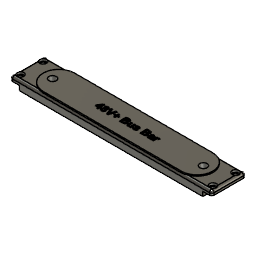
Compartment Mount (Autodesk Fusion 360 archive; units mm, degrees)
design "Upper Platform"
part number: 2026-01-22-12-11-46-373
Autodesk Fusion 360 part; units mm, degrees
sketch "Base" plane through (0, 0, 0) normal (0, 0, 1) x (1, 0, 0)
  line L0 (89, 15) -> (-89, 15)
  line L1 (-89, 15) -> (-89, -15)
  line L2 (-89, -15) -> (89, -15)
  line L3 (89, -15) -> (89, 15)
  line L4 (89, 15) -> (-89, -15) construction
  line L5 (-89, 15) -> (89, -15) construction
  line L6 (81, 15) -> (-81, 15)
  line L7 (-81, 15) -> (-81, -15)
  line L8 (-81, -15) -> (81, -15)
  line L9 (81, -15) -> (81, 15)
  line L10 (81, 15) -> (-81, -15) construction
  line L11 (-81, 15) -> (81, -15) construction
  dimension "d1" = 178
  dimension "d2" = 30
  dimension "d3" = 162
  constraint horizontal L0
  constraint perpendicular L0 L1
  constraint parallel L0 L2
  constraint parallel L1 L3
  constraint coincident L4 origin
  constraint coincident L5 origin
  constraint horizontal L6
  constraint perpendicular L6 L7
  constraint parallel L6 L8
  constraint parallel L7 L9
  constraint coincident L10 origin
  constraint coincident L11 origin
  measures "d1" distance of L1.end L2.end
  measures "d2" distance of L0.end L1.end
  measures "d3" distance of L7.end L8.end
extrude "Extrude1" add sketch "Base" against normal blind 4 contours L0 L2 L6 L7 L8 L9
extrude "Extrude2" add sketch "Base" along normal blind 4
sketch "Mounting Holes" plane through (0, 0, 4) normal (0, 0, 1) x (-1, 0, 0)
  line L0 (89, 15) -> (-89, 15)
  line L1 (-89, 15) -> (-89, -15)
  line L2 (-89, -15) -> (89, -15)
  line L3 (89, -15) -> (89, 15)
  line L4 (61, 14) -> (-61, 14)
  line L5 (-61, -14) -> (61, -14)
  line L6 (75, 14) -> (-75, -14) construction
  line L7 (-75, 14) -> (75, -14) construction
  arc A0 (61, -14) -> (75, 0) centre (61, 0) ccw
  arc A1 (75, 0) -> (61, 14) centre (61, 0) ccw
  arc A2 (-61, 14) -> (-75, 0) centre (-61, 0) ccw
  arc A3 (-75, 0) -> (-61, -14) centre (-61, 0) ccw
  circle A4 centre (85, -10) radius 2
  circle A5 centre (85, -10) radius 3
  circle A6 centre (-85, -10) radius 3
  circle A7 centre (-85, -10) radius 2
  circle A8 centre (85, 10) radius 3
  circle A9 centre (85, 10) radius 2
  circle A10 centre (-85, 10) radius 3
  circle A11 centre (-85, 10) radius 2
  dimension "d8" = 150
  dimension "d9" = 28
  dimension "d10" = 14
  dimension "d11" = 14
  dimension "d12" = 14
  dimension "d13" = 14
  dimension "d14" = 4
  dimension "d15" = 6
  dimension "d18" = -170
  dimension "d19" = 20
  constraint horizontal L4
  constraint parallel L4 L5
  constraint coincident L6 origin
  constraint coincident L7 origin
  constraint coincident L7.end L5
  constraint tangent L5 A0
  constraint coincident L6.start L4
  constraint tangent L4 A1
  constraint coincident A0.end A1.start
  constraint coincident L7.start L4
  constraint tangent L4 A2
  constraint coincident L6.end L5
  constraint tangent L5 A3
  constraint coincident A2.end A3.start
  constraint concentric A4 A5
  measures "d8" distance of L6.end L7.end
  measures "d9" distance of L7.start L6.end
  measures "d10" radius of A0
  measures "d11" radius of A1
  measures "d12" radius of A2
  measures "d13" radius of A3
  measures "d14" diameter of A4
  measures "d15" diameter of A5
extrude "Extrude3" cut sketch "Mounting Holes" against normal blind 2 contours A5 | A6 | A8 | A10
extrude "Extrude4" cut 4 faces at (85.7854, 10.4534, 4) (85.7854, -9.5466, 4) (-84.2146, 10.4534, 4) (-84.2146, -9.5466, 4) along direction (0, 0, -1) through all
extrude "Extrude5" add sketch "Mounting Holes" along normal blind 1 contours L4 L5 A0 A1 A2 A3
sketch "48V+BusBar Mount" plane through (0, 0, 5) normal (0, 0, 1) x (-1, 0, 0)
  arc A0 (-61, 14) -> (-61, -14) centre (-61, 0) ccw
  line L0 (-61, -14) -> (61, -14)
  arc A1 (61, -14) -> (61, 14) centre (61, 0) ccw
  line L1 (61, 14) -> (-61, 14)
  line L2 (-61, -14) -> (61, -14)
  circle A2 centre (66.6, 0) radius 3.25
  circle A3 centre (-66.6, 0) radius 3.25
  line L3 (60, 10) -> (-60, 10) construction
  line L4 (-60, 10) -> (-60, -10) construction
  line L5 (-60, -10) -> (60, -10) construction
  line L6 (60, -10) -> (60, 10) construction
  point P0 (66.6, 0)
  point P1 (75, 0)
  point P2 (-66.6, 0)
  dimension "d25" = 8.4
  dimension "d26" = 14
  dimension "d27" = 6.5
  dimension "d30" = -133.2
  dimension "d31" = 0
  dimension "d32" = 6
  dimension "d33" = 0
  text T0 "48V+ Bus Bar" font "Arial" height 6 bold align centre middle in box 120 x 20 at (60, 10) x (-1, 0) y (0, -1) spacing 1 kerned
  constraint coincident P0 A2.centre
  measures "d25" distance of P0 P1
  measures "d26" distance of P0 L2
  measures "d27" diameter of A2
extrude "Extrude6" cut sketch "48V+BusBar Mount" against normal blind 7 contours A2 | A3
extrude "Extrude7" cut sketch "48V+BusBar Mount" against normal blind 1 text T0
fillet "Fillet1" radius 2 4 edges at (-89, -15, 2) (89, -15, 2) (89, 15, 2) (-89, 15, 2)
fillet "Fillet2" radius 2 8 edges at (-88.4142, -14.4142, 4) (0, -15, 4) (88.4142, -14.4142, 4) (89, 0, 4) (88.4142, 14.4142, 4) (0, 15, 4) (-88.4142, 14.4142, 4) (-89, 0, 4)
equation "d33 = '48V+ Bus Bar'"
named bodies: "Body1"

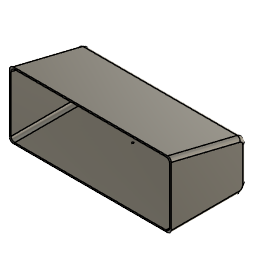
design "Right Dash Compartment"
part number: 2026-01-22-12-27-07-009
Autodesk Fusion 360 part; units mm, degrees
sketch "Base" plane through (0, 0, 0) normal (0, 0, 1) x (1, 0, 0)
  line L0 (215, 100) -> (-215, 100)
  line L1 (-215, 100) -> (-215, -100)
  line L2 (-215, -100) -> (215, -100)
  line L3 (215, -100) -> (215, 100)
  line L4 (215, 100) -> (-215, -100) construction
  line L5 (-215, 100) -> (215, -100) construction
  dimension "d1" = 430
  dimension "d2" = 200
  constraint horizontal L0
  constraint perpendicular L0 L1
  constraint parallel L0 L2
  constraint parallel L1 L3
  constraint coincident L4 origin
  constraint coincident L5 origin
  measures "d1" distance of L1.end L2.end
  measures "d2" distance of L0.end L1.end
extrude "Extrude1" add sketch "Base" along normal blind 4
sketch "Back" plane through (0, 0, 0) normal (0, 1, 0) x (1, 0, 0)
  line L0 (-215, 0, 100) -> (215, 0, 100)
  line L1 (215, 0, 100) -> (215, -130, 100)
  line L2 (215, -130, 100) -> (-215, -130, 100)
  line L3 (-215, -130, 100) -> (-215, 0, 100)
  dimension "d5" = 130
extrude "Extrude2" add sketch "Back" along normal blind 4 contours L0 L1 L2 L3 in plane through (0, 100, 0) normal (0, 1, 0)
sketch "Right Side" plane through (215, 0, 0) normal (1, 0, 0) x (0, 1, 0)
  line L0 (-100, 0) -> (100, 0)
  line L1 (100, 0) -> (104, 0)
  line L2 (104, 0) -> (104, 130)
  line L3 (100, 4) -> (-100, 4)
  line L4 (-100, 4) -> (-100, 0)
  line L5 (-100, 0) -> (104, 0)
  line L6 (104, 0) -> (104, 130)
  line L7 (-100, 130) -> (-100, 0)
  line L8 (-100, 130) -> (-100, 180)
  line L9 (-100, 180) -> (104, 130)
  line L10 (100, 126.862) -> (-100, 175.8816)
  line L11 (100, 126.862) -> (104, 126.862)
  line L12 (104, 130) -> (104, 126.862)
  line L13 (100, 126.862) -> (100, 4)
  constraint horizontal L5
  constraint vertical L6
  constraint vertical L7
  constraint coincident L2.end L6.end
  constraint coincident L0.start L4.end
  constraint coincident L8 L10.end
  constraint coincident L2 L11.end
  constraint perpendicular L2 L11
  constraint coincident L3.start L13.end
  constraint perpendicular L3 L13
extrude "Extrude3" add sketch "Right Side" along normal blind 4
extrude "Extrude4" add sketch "Right Side" against normal blind 430 contours L2 L6 L8 L9 L10 L11 L12
sketch "Left Side" plane through (-215, 0, 0) normal (-1, 0, 0) x (0, -1, 0)
  line L0 (-104, 130) -> (-104, 0)
  line L1 (-104, 0) -> (100, 0)
  line L2 (100, 0) -> (100, 4)
  line L3 (100, 4) -> (-100, 4)
  line L4 (-100, 4) -> (-100, 126.862)
  line L5 (-100, 126.862) -> (100, 175.8816)
  line L6 (100, 175.8816) -> (100, 180)
  line L7 (100, 180) -> (-104, 130)
  line L8 (100, 0) -> (100, 180)
  constraint coincident L1.end L2.start
  constraint coincident L6.end L7.start
extrude "Extrude5" add sketch "Left Side" along normal blind 4
fillet "Fillet1" radius 20 2 edges at (0, 100, 4) (0, 100, 126.862)
fillet "Fillet2" radius 10 10 edges at (215, -10, 4) (215, 94.1421, 9.8579) (215, 100, 67.586) (215, 95.7356, 123.5166) (215, -7.6195, 153.2393) (-215, -7.6195, 153.2393) (-215, 95.7356, 123.5166) (-215, 100, 67.586) (-215, 94.1421, 9.8579) (-215, -10, 4)
fillet "Fillet3" radius 20 7 edges at (217, 104, 0) (-2, 104, 0) (217, 104, 0) (-2, 104, 0) (-2, 104, 130) (217, 104, 130) (-2, 104, 130)
fillet "Fillet4" radius 10 10 edges at (219, -8, 0) (219, 98.1421, 5.8579) (219, 104, 67.155) (219, 99.7356, 126.6546) (219, -5.6195, 156.8675) (-219, -5.6195, 156.8675) (-219, 99.7356, 126.6546) (-219, 104, 67.155) (-219, 98.1421, 5.8579) (-219, -8, 0)
sketch "Mounting Holes" plane through (0, 0, 4) normal (0, 0, 1) x (-1, 0, 0)
  line L0 (205, -80) -> (205, 100)
  line L1 (205, 100) -> (-205, 100)
  line L2 (-205, 100) -> (-205, -80)
  line L3 (-205, -80) -> (205, -80)
  line L4 (-175, 100) -> (45, 100)
  line L5 (45, 100) -> (45, -60)
  line L6 (45, -60) -> (-175, -60)
  line L7 (-175, -60) -> (-175, 100)
  circle A0 centre (-175, -60) radius 2.75
  circle A1 centre (45, -60) radius 2.75
  dimension "d23" = 220
  dimension "d24" = 160
  dimension "d25" = 5.5
  dimension "d26" = 5.5
  constraint horizontal L4
  constraint vertical L5
  constraint horizontal L6
  constraint vertical L7
  constraint coincident L1 L4.start
  constraint coincident L6.end L7.start
  constraint coincident L5.end L6.start
  measures "d23" distance of L4.start L4.end
  measures "d24" distance of L4.start L6.end
  measures "d25" diameter of A0
  measures "d26" diameter of A1
extrude "Extrude6" cut sketch "Mounting Holes" against normal through all contours L5 L6 A1 | L5 L6 A1 | L6 L7 A0 | L6 L7 A0
